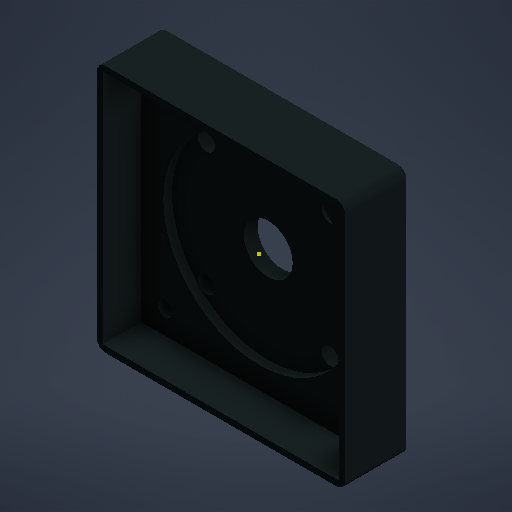
# Autodesk Inventor part: GEARBOX-SUPPORT
Saved by Autodesk Inventor 2025.3 (Build 293356030, 356C)
## iProperties
Created: 2025-10-20
Part Number: GEARBOX-SUPPORT
Material: Generic
Document SubType Name: Modeling
Designer: lstk1ng
Density: 1 g/cm^3
Appearance: Gray
Author: lstk1ng
Autodesk Inventor part; units mm, degrees
ref_plane "YZ Plane" through (0, 0, 0) normal (1, 0, 0) x (0, 1, 0)
ref_plane "XZ Plane" through (0, 0, 0) normal (0, 1, 0) x (-1, 0, 0)
ref_plane "XY Plane" through (0, 0, 0) normal (0, 0, 1) x (1, 0, 0)
sketch "Sketch1" plane through (0, 0, 0) normal (0, 0, 1) x (1, 0, 0)
  line L0 (71, 71) -> (-71, 71)
  line L1 (-71, 71) -> (-71, -71)
  line L2 (-71, -71) -> (71, -71)
  line L3 (71, -71) -> (71, 71)
  point P0 (0, 0)
  constraints: 8 end point
extrude "Extrusion1" add sketch "Sketch1" along normal blind 35
fillet "Fillet1" radius 5 4 edges at (-71, -71, 17.5) (-71, 71, 17.5) (71, 71, 17.5) (71, -71, 17.5)
sketch "Sketch6" plane through (0, 0, 35) normal (0, 0, 1) x (1, 0, 0)
  line L0 (-67.5, -67.5) -> (67.5, -67.5)
  line L1 (67.5, -67.5) -> (67.5, 67.5)
  line L2 (67.5, 67.5) -> (-67.5, 67.5)
  line L3 (-67.5, 67.5) -> (-67.5, -67.5)
  line L4 (-67.5, -67.5) -> (67.5, 67.5) construction
  line L5 (67.5, -67.5) -> (-67.5, 67.5) construction
  point P0 (0, 0)
  dimension "d26" = 135
  dimension "d27" = 135
  constraints: 12 end point, 2 midpoint, 2 parallel, 1 horizontal, 1 perpendicular
  measures "d26" distance of L2.end L1.end
  measures "d27" distance of L1.end L0.end
extrude "Extrusion6" cut sketch "Sketch6" against normal blind 22
sketch "Sketch7" plane through (0, 0, 13) normal (0, 0, 1) x (1, 0, 0)
  point P0 (0, 0)
sketch "Sketch8" plane through (0, 0, 13) normal (0, 0, 1) x (1, 0, 0)
  circle A0 centre (0, 0) radius 55
  dimension "d30" = 110
  constraints: 1 centre point, 1 coincident
  measures "d30" diameter of A0
extrude "Extrusion7" cut sketch "Sketch8" against normal blind 5
sketch "Sketch9" plane through (0, 0, 8) normal (0, 0, 1) x (1, 0, 0)
  circle A0 centre (0, 0) radius 14
  dimension "d33" = 28
  constraints: 1 centre point, 1 coincident
  measures "d33" diameter of A0
extrude "Extrusion8" cut sketch "Sketch9" against normal through all
sketch "Sketch10" plane through (0, 0, 0) normal (0, 0, -1) x (-1, 0, 0)
  circle A0 centre (0, 0) radius 76.4 construction
  line L0 (0, 0) -> (54.023, -54.023) construction
  line L1 (0, 0) -> (76.4, 0) construction
  line L2 (0, 0) -> (0, -71) construction
  line L3 (66, -71) -> (-66, -71) projected
  line L4 (0, 0) -> (-76.4, 0) construction
  line L5 (-67.5, 67.5) -> (-67.5, -67.5) projected
  circle A1 centre (54.023, -54.023) radius 4.25
  circle A2 centre (-54.023, -54.023) radius 4.25
  circle A3 centre (54.023, 54.023) radius 4.25
  circle A4 centre (-54.023, 54.023) radius 4.25
  circle A5 centre (0, 0) radius 50 construction
  circle A6 centre (35.3553, -35.3553) radius 4.85
  circle A7 centre (-35.3553, -35.3553) radius 4.85
  circle A8 centre (35.3553, 35.3553) radius 4.85
  circle A9 centre (-35.3553, 35.3553) radius 4.85
  dimension "d41" = 100
  dimension "d36" = 152.8
  dimension "d37" = 45
  dimension "d38" = 8.5
  dimension "d42" = 9.7
  constraints: 9 centre point, 8 end point, 6 symmetric about line, 3 coincident, 2 horizontal, 2 point on circle, 1 equal length, 1 midpoint, 1 point on line, 10 other
  measures "d36" diameter of A0
  measures "d37" angle of L0 L1
  measures "d38" diameter of A1
  measures "d42" diameter of A6
extrude "Extrusion9" cut sketch "Sketch10" against normal through all
sketch "Sketch12" plane through (0, 0, 0) normal (0, 0, -1) x (-1, 0, 0)
  circle A0 centre (35.3553, -35.3553) radius 4.85 projected
  circle A1 centre (35.3553, 35.3553) radius 4.85 projected
  circle A2 centre (-35.3553, 35.3553) radius 4.85 projected
  circle A3 centre (-35.3553, -35.3553) radius 4.85 projected
  circle A4 centre (35.3553, -35.3553) radius 6.85
  circle A5 centre (-35.3553, -35.3553) radius 6.85
  circle A6 centre (-35.3553, 35.3553) radius 6.85
  circle A7 centre (35.3553, 35.3553) radius 6.85
  point P0 (0, 0)
  constraints: 4 centre point
extrude "Extrusion10" add sketch "Sketch12" along normal blind 5
body "Solid1"
